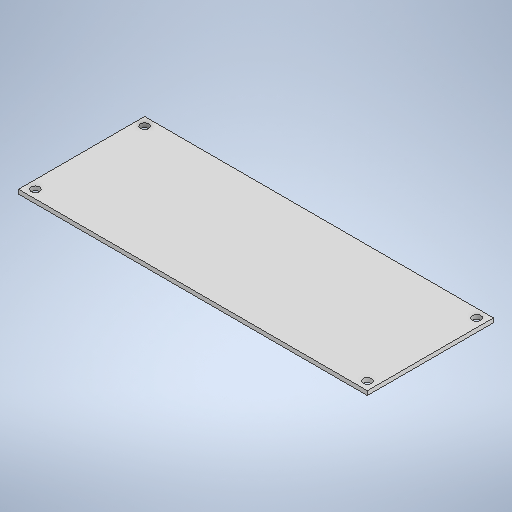
# Autodesk Inventor part: PCB
Saved by Autodesk Inventor 2025.2 (Build 292293000, 293)
## iProperties
Created: 2026-03-13
Part Number: PCB
Material: Genérico
Document SubType Name: Modeling
Designer: Periscopio
Density: 1 g/cm^3
Appearance: Valor por defecto
Author: Periscopio
Autodesk Inventor part; units mm, degrees
ref_plane "YZ Plane" through (0, 0, 0) normal (1, 0, 0) x (0, 1, 0)
ref_plane "XZ Plane" through (0, 0, 0) normal (0, 1, 0) x (-1, 0, 0)
ref_plane "XY Plane" through (0, 0, 0) normal (0, 0, 1) x (1, 0, 0)
sketch "Boceto1" plane through (0, 0, 0) normal (0, 1, 0) x (-1, 0, 0)
  line L0 (41.5, 15) -> (-41.5, 15)
  line L1 (-41.5, 15) -> (-41.5, -15)
  line L2 (-41.5, -15) -> (41.5, -15)
  line L3 (41.5, -15) -> (41.5, 15)
  line L4 (41.5, 15) -> (-41.5, -15) construction
  line L5 (-41.5, 15) -> (41.5, -15) construction
  point P0 (0, 0)
  dimension "d0" = 83
  dimension "d1" = 30
  constraints: 12 end point, 2 midpoint, 2 parallel, 1 horizontal, 1 perpendicular
  measures "d0" distance of L2.end L1.end
  measures "d1" distance of L1.end L0.end
extrude "Extrusión1" add sketch "Boceto1" along normal blind 1
sketch "Boceto2" plane through (0, 1, 0) normal (0, 1, 0) x (1, 0, 0)
  line L0 (41.5, 15) -> (-41.5, 15) projected
  line L1 (-41.5, 15) -> (-18.7131, 15) construction
  circle A0 centre (-39.5, 13) radius 1
  circle A1 centre (39.5, 13) radius 1
  circle A2 centre (-39.5, -13) radius 1
  circle A3 centre (39.5, -13) radius 1
  point P0 (0, 0)
  dimension "d5" = 2
  dimension "d6" = 2
  constraints: 4 centre point, 2 end point, 1 horizontal
  measures "d5" diameter of A0
  measures "d6" distance from line of L0 A0.centre
extrude "Extrusión2" cut sketch "Boceto2" against normal through all
